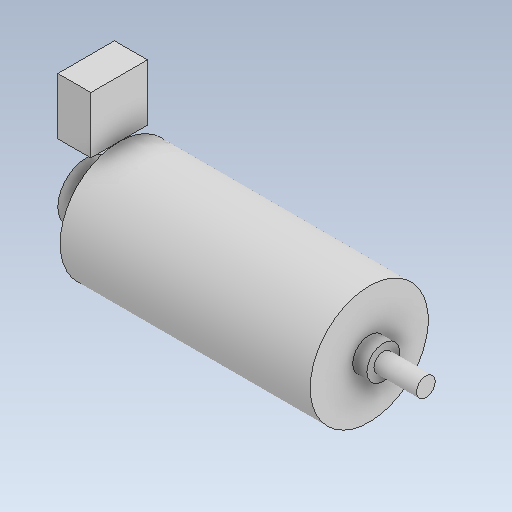
# Autodesk Inventor part: 02_Motor
Saved by Autodesk Inventor 2021 (Build 250183000, 183)
## iProperties
Created: 2021-03-20
Part Number: 02_Motor
Material: Generisch
Document SubType Name: Modeling
Designer: User
Density: 1 g/cm^3
Appearance: Vorgabe
Author: User
Autodesk Inventor part; units mm, degrees
ref_plane "YZ Plane" through (0, 0, 0) normal (1, 0, 0) x (0, 1, 0)
ref_plane "XY Plane" through (0, 0, 0) normal (0, 0, 1) x (1, 0, 0)
derived "00_Mastersketch.ipt"
sketch "02_motorSketch" plane through (67, -17.95, 0) normal (0, 1, 0) x (-1, 0, 0)
  line L0 (3, 12.5) -> (3, -12.5) construction
  line L1 (3, -12.5) -> (56, -12.5) construction
  line L2 (56, -12.5) -> (56, 12.5) construction
  line L3 (56, 12.5) -> (3, 12.5) construction
  line L4 (56, 6) -> (63, 6) construction
  line L5 (63, 6) -> (63, -6) construction
  line L6 (63, -6) -> (56, -6) construction
  line L7 (63, 0) -> (-9, 0)
  line L8 (63, 0) -> (63, 6)
  line L9 (63, 6) -> (56, 6)
  line L10 (56, 12.5) -> (56, 6)
  line L11 (56, 12.5) -> (3, 12.5)
  line L12 (0, 3.5) -> (3, 3.5) construction
  line L13 (0, 2) -> (0, 3.5) construction
  line L14 (-9, 2) -> (0, 2) construction
  line L15 (-9, -2) -> (-9, 2) construction
  line L16 (3, 12.5) -> (3, 3.5)
  line L17 (0, 3.5) -> (3, 3.5)
  line L18 (0, 3.5) -> (0, 2)
  line L19 (0, 2) -> (-9, 2)
  line L20 (-9, 2) -> (-9, 0)
  point P0 (67, 0)
  point P1 (-78.175, 0)
  point P2 (-66.175, 12.5)
revolve "Umdrehung2" add sketch "02_motorSketch" angle 360 about axis through (4, -17.95, 0) along (1, 0, 0)
ref_plane "Arbeitsebene1" through (37.5, -5.45, 0) normal (0, 1, 0) x (-1, 0, 0)
sketch "Skizze2" plane through (37.5, -5.45, 0) normal (0, 1, 0) x (-1, 0, 0)
  line L0 (26.5, 6) -> (33.5, 6) projected
  line L1 (33.5, -6) -> (33.5, 6) projected
  line L2 (26.5, -6) -> (33.5, -6) projected
  line L3 (26.5, -6) -> (26.5, 6) projected
  point P0 (37.5, 0)
extrude "Extrusion1" add sketch "Skizze2" along normal blind 12
